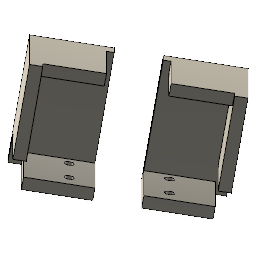
Top Corner Brackets (Autodesk Fusion 360 design; units mm, degrees)
Autodesk Fusion 360 part; units mm, degrees
note: some values were not read from the file. Set by a fixed rule: which sketch regions a step uses.
sketch "Sketch1" plane through (0, 0, 0) normal (0, 0, 1) x (1, 0, 0)
  line L0 (12.7, 12.7) -> (-12.7, 12.7)
  line L1 (-12.7, 12.7) -> (-12.7, -12.7)
  line L2 (-12.7, -12.7) -> (12.7, -12.7)
  line L3 (12.7, -12.7) -> (12.7, 12.7)
  line L4 (12.7, 12.7) -> (-12.7, -12.7) construction
  line L5 (-12.7, 12.7) -> (12.7, -12.7) construction
  line L6 (-12.7, 12.7) -> (12.7, 12.7)
  line L7 (12.7, 12.7) -> (12.7, 8.7)
  line L8 (12.7, 8.7) -> (-12.7, 8.7)
  line L9 (-12.7, 8.7) -> (-12.7, 12.7)
  line L10 (12.7, 12.7) -> (8.7, 12.7)
  line L11 (8.7, 12.7) -> (8.7, -12.7)
  line L12 (8.7, -12.7) -> (12.7, -12.7)
  line L13 (12.7, -12.7) -> (12.7, 12.7)
  circle A0 centre (-5, 5) radius 1.5
  circle A1 centre (-5, -7) radius 1.5
  dimension "d1" = 25.4
  dimension "d2" = 25.4
  dimension "d5" = 4
  dimension "d6" = 4
  dimension "d17" = 3
  dimension "d18" = 3
  constraint perpendicular L0 L1
  constraint parallel L0 L2
  constraint parallel L1 L3
  constraint horizontal L0
  constraint coincident L4 origin
  constraint coincident L5 origin
  constraint horizontal L6
  constraint vertical L7
  constraint horizontal L8
  constraint vertical L9
  constraint horizontal L10
  constraint vertical L11
  constraint horizontal L12
  constraint vertical L13
  measures "d1" distance of L0.end L1.end
  measures "d2" distance of L1.end L2.end
  measures "d5" distance of L0.end L8.end
  measures "d6" distance of L0.start L10.end
  measures "d17" diameter of A0
  measures "d18" diameter of A1
extrude "Extrude1" add sketch "Sketch1" along normal blind 4 makes body 1
extrude "Extrude2" add sketch "Sketch1" along normal blind 39.25 contours L0 L3 L6 L7 L8 L10 L11 L13 | L0 L1 L6 L8 L9 L11 bodies 1
extrude "Extrude3" add sketch "Sketch1" along normal blind 39.25 contours L2 L3 L8 L11 L12 L13 bodies 1
extrude "Extrude4" cut sketch "Sketch1" along normal blind 9 contours L2 L3 L8 L11 L12 L13 bodies 1
sketch "Sketch2" plane through (0, 0, 39.25) normal (0, 0, 1) x (1, 0, 0)
  line L0 (12.7, 12.7) -> (-12.7, 12.7)
  line L1 (-12.7, 12.7) -> (-12.7, 8.7)
  line L2 (-12.7, 8.7) -> (8.7, 8.7)
  line L3 (12.7, -12.7) -> (12.7, 12.7)
  line L4 (8.7, 8.7) -> (-10.35, 8.7)
  line L5 (-10.35, 8.7) -> (-10.35, -10.35)
  line L6 (-10.35, -10.35) -> (8.7, -10.35)
  line L7 (8.7, -10.35) -> (8.7, 8.7)
  line L8 (8.7, 8.7) -> (8.7, -12.7)
  line L9 (8.7, -12.7) -> (12.7, -12.7)
  dimension "d13" = 19.05
  dimension "d14" = 19.05
  constraint horizontal L4
  constraint vertical L5
  constraint horizontal L6
  constraint vertical L7
  constraint coincident L2.end L4.start
  measures "d13" distance of L2.end L4.end
  measures "d14" distance of L2.end L6.end
extrude "Extrude5" add sketch "Sketch2" against normal blind 4 contours L2 L4 L5 L6 L7 L8 bodies 1
ref_plane "WorkPlane1" through (-20, 0, 0) normal (1, 0, 0) x (0, 1, 0)
mirror "Mirror1" about plane through (-20, 0, 0) normal (1, 0, 0) of bodies 1 makes body 2
